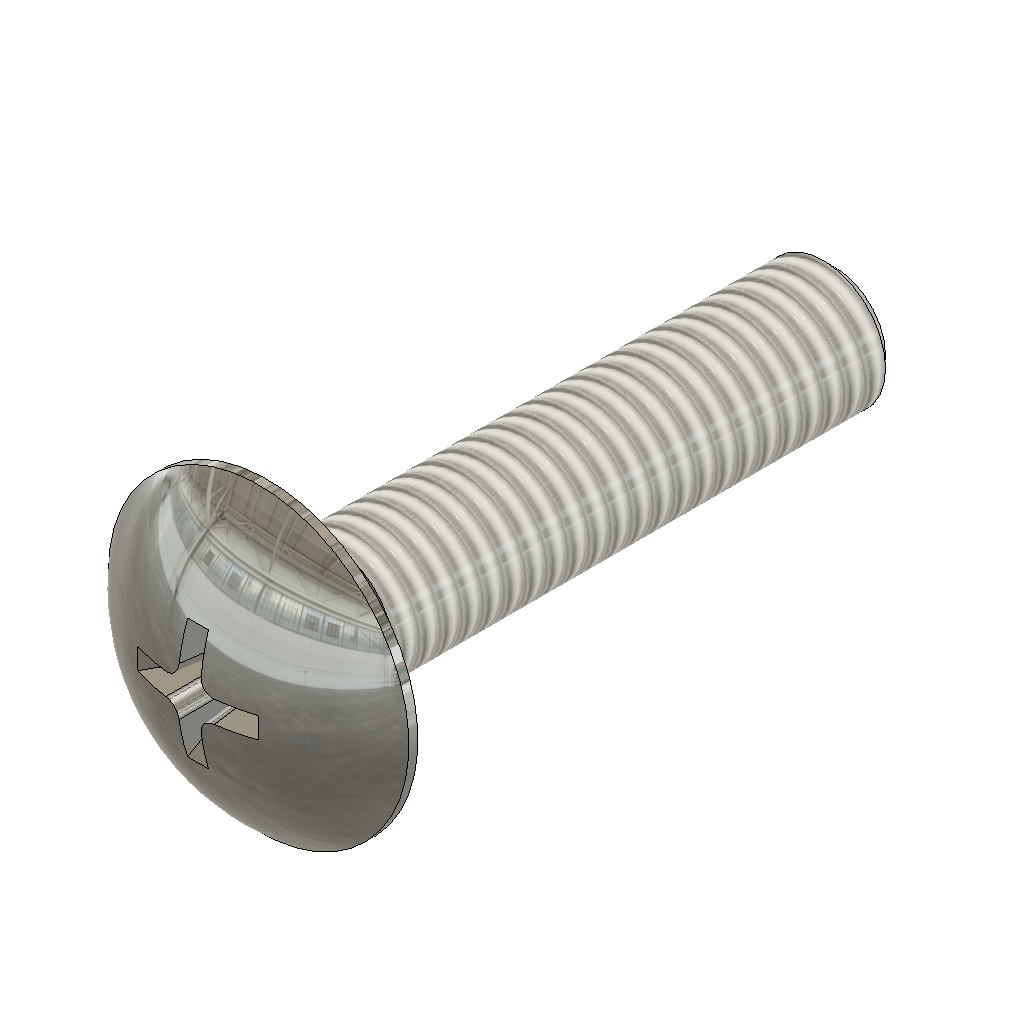
SdvxPanel (Assembly) (Autodesk Fusion 360 archive; units mm, degrees)
design "Truss Head Screw JIS B 1111 - M4.5x20 Steel 4.6 Chrome"
description: Truss Head Screw JIS B 1111 - M4.5x20
part number: THS JIS B 1111 - M4.5x20 Steel 4.6 Chrome
Autodesk Fusion 360 part; units mm, degrees
(part 1 of 4)
sketch "Sketch1" plane through (0, 0, 0) normal (0, 1, 0) x (1, 0, 0)
  line L0 (-2.25, 2.25) -> (-2.25, 20)
  line L1 (-2.25, 20) -> (0, 20)
  line L2 (0, 20) -> (0, -2.8)
  line L3 (-1.9125, 0) -> (-5.3, 0)
  line L4 (-5.3, 0) -> (-5.3, -0.3181)
  arc A0 (-5.3, -0.3181) -> (0, -2.8) centre (0, 4.1) ccw
  line L5 (-2.25, 2.25) -> (-1.9125, 2.25)
  line L6 (-1.9125, 2.25) -> (-1.9125, 0)
  dimension "d9" = 4.5
  dimension "d66" = 10.6
  dimension "d76" = 3.825
  dimension "d78" = 2.25
  dimension "d98" = 2.8
  dimension "d100" = 20
  constraint perpendicular L0 L1
  constraint perpendicular L0 L3
  constraint coincident origin L3
  constraint vertical L0
  constraint vertical L2
  constraint vertical L4
  constraint coincident L2 A0.centre
  constraint coincident L2.end A0.end
  constraint coincident L3.start L6.end
  constraint coincident origin L2
  measures "d78" distance of L3 L5
  measures "d98" distance of L3 L2.end
  measures "d100" distance of origin L1
revolve "Revolve1" add sketch "Sketch1" angle 360 about axis through (0, 0, -20) along (0, 0, 1) makes body 1
ref_plane "WorkPlane1" through (0, 0, 2.8) normal (0, 0, 1) x (1, 0, 0)
sketch "Sketch2" plane through (0, 0, 2.8) normal (0, 0, 1) x (1, 0, 0)
  line L0 (-0.3917, 0.3917) -> (-2.35, 0.3917)
  line L1 (-0.3917, -0.3917) -> (-2.35, -0.3917)
  line L2 (-2.35, 0.3917) -> (-2.35, -0.3917)
  line L3 (-0.3917, -0.3917) -> (-0.3917, -2.35)
  line L4 (-0.3917, -2.35) -> (0.3917, -2.35)
  line L5 (0.3917, -0.3917) -> (0.3917, -2.35)
  line L6 (0.3917, -0.3917) -> (2.35, -0.3917)
  line L7 (2.35, -0.3917) -> (2.35, 0.3917)
  line L8 (0.3917, 0.3917) -> (2.35, 0.3917)
  line L9 (0.3917, 0.3917) -> (0.3917, 2.35)
  line L10 (0.3917, 2.35) -> (-0.3917, 2.35)
  line L11 (-0.3917, 0.3917) -> (-0.3917, 2.35)
  dimension "d94" = 360
  dimension "d101" = 0.7833
  dimension "d102" = 4.7
  constraint horizontal L0
  constraint vertical L0.start L1.start
  constraint coincident L0.start L11.start
  constraint vertical L2
  measures "d101" distance of L0 L1
  measures "d102" distance of L2 L7
extrude "Extrude1" add sketch "Sketch2" against normal blind 2.53 draft -4 separate body makes body 2
draft "Draft1" angle -30 neutral plane through (0, 0, 2.8) pull (0, 0, 1) 4 faces at (-2.291, -0.0716, 1.9567) (0.0716, -2.291, 1.9567) (2.291, 0.0716, 1.9567) (0.0716, 2.291, 1.9567) on bodies 2
fillet "Fillet3" radius 0.47 4 edges at (-0.3032, 0.3032, 1.535) (0.3032, 0.3032, 1.535) (0.3032, -0.3032, 1.535) (-0.3032, -0.3032, 1.535) on bodies 2
combine "Combine1" operation cut target body 1 tool bodies 2
thread "Thread1" "ISO Metric profile 4.5 M4.5x0.75 M4.5x0.75 6g" major diameter 4.408 minor diameter 3.5525 pitch 0.75 angle 60 resizes the face on face at (-2.2388, 0.224, -8.1667) on bodies 1
sketch "Sketch6" plane through (0, 0, 0) normal (0, 1, 0) x (1, 0, 0)
  line L0 (-1.8, 20) -> (-2.295, 20)
  line L1 (-2.295, 20) -> (-2.295, 19.505)
  line L2 (-2.295, 19.505) -> (-1.8, 20)
  point P0 (0, 20)
  dimension "d83" = 45
  dimension "d85" = 2.295
  dimension "d103" = 0.495
  constraint horizontal L0
  constraint perpendicular L0 L1
  constraint coincident L0 P0
  measures "d83" angle of L1 L2
  measures "d85" distance of origin L1
  measures "d103" distance of L0 L1.end
revolve "Revolve3" cut sketch "Sketch6" angle 360 about axis through (0, 0, 1.75) along (0, 0, 1) bodies 1
equation "d9 = adsk_nomdia"
equation "adsk_nomlen = 20.00 mm"
equation "adsk_headh = 2.80 mm"
equation "adsk_headdia = 10.60 mm"
equation "adsk_nomdia = 4.50 mm"
equation "adsk_phildia = 4.70 mm"
equation "adsk_phildepth = 2.53 mm"
equation "d66 = adsk_headdia"
equation "d71 = adsk_headh"
equation "adsk_thrlen = 17.75 mm"
equation "d76 = adsk_nomdia * 0.85"
equation "d78 = adsk_nomlen - adsk_thrlen"
equation "d85 = adsk_nomdia * 0.51"
equation "adsk_ovalrad = 6.90 mm"
equation "d97 = adsk_phildia * 0.1"
equation "d98 = adsk_headh"
equation "d100 = adsk_nomlen"
equation "d101 = adsk_phildia / 6"
equation "d102 = adsk_phildia"
equation "d103 = adsk_nomdia * 0.1 + ( adsk_nomdia * 0.01 )"

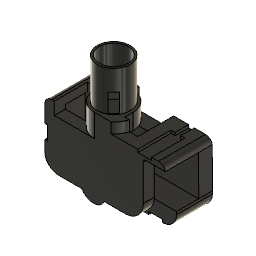
design "OBSA-LHS1F"
Autodesk Fusion 360 part; units mm, degrees
sketch "Sketch1" plane through (0, 0, 0) normal (0, 1, 0) x (1, 0, 0) in component "housing"
  line L0 (21.875, 5.25) -> (21.875, 6.25)
  line L1 (21.875, 11.25) -> (-21.875, -11.25) construction
  line L2 (-21.875, 11.25) -> (21.875, -11.25) construction
  line L3 (-0.275, 11.25) -> (-0.275, 13.75) construction
  line L4 (-0.275, 13.75) -> (-8.375, 13.75) construction
  line L5 (-8.375, 13.75) -> (-8.375, 11.25) construction
  arc A0 (21.875, 6.25) -> (16.875, 11.25) centre (16.875, 6.25) ccw
  arc A1 (-16.875, 11.25) -> (-21.875, 6.25) centre (-16.875, 6.25) ccw
  line L6 (-18.375, -11.25) -> (-18.375, -6.75)
  arc A2 (-21.875, -8.75) -> (-19.375, -11.25) centre (-19.375, -8.75) ccw
  line L7 (-18.375, -6.75) -> (-6.875, -6.75)
  line L8 (-6.875, -6.75) -> (-6.875, -11.25)
  line L9 (21.875, 5.25) -> (13.8245, 5.25)
  arc A3 (19.375, -11.25) -> (21.8245, -9.25) centre (19.375, -8.75) ccw
  line L10 (21.8245, -9.25) -> (14.8245, -9.25)
  line L11 (13.8245, -8.25) -> (13.8245, 5.25)
  line L12 (-19.375, -11.25) -> (-18.375, -11.25)
  arc A4 (-0.275, 11.25) -> (-8.375, 11.25) centre (-4.325, 9.2195) ccw
  line L13 (-8.375, 11.25) -> (-16.875, 11.25)
  line L14 (16.8245, -11.25) -> (16.8245, -10.25)
  line L15 (16.8245, -10.25) -> (11.8245, -10.25)
  line L16 (11.8245, -10.25) -> (11.8245, -11.25)
  line L17 (7.8245, -11.25) -> (11.8245, -11.25)
  line L18 (16.8245, -11.25) -> (19.375, -11.25)
  line L19 (-21.875, -2.5) -> (-20.875, -2.5)
  line L20 (-20.875, -2.5) -> (-20.875, 2.5)
  line L21 (-20.875, 2.5) -> (-21.875, 2.5)
  line L22 (-21.875, 6.25) -> (-21.875, 2.5)
  line L23 (-21.875, -2.5) -> (-21.875, -8.75)
  line L24 (-21.4773, 11.25) -> (-21.4773, 0) construction
  line L25 (-20.875, 0) -> (-22.0795, 0) construction
  line L26 (-21.4773, -11.25) -> (-21.4773, 0) construction
  arc A5 (13.8245, -8.25) -> (14.8245, -9.25) centre (14.8245, -8.25) ccw
  line L27 (11.8245, 11.25) -> (11.8245, 10.25)
  line L28 (11.8245, 10.25) -> (16.8245, 10.25)
  line L29 (16.8245, 10.25) -> (16.8245, 11.25)
  line L30 (16.875, 11.25) -> (16.8245, 11.25)
  line L31 (11.8245, 11.25) -> (-0.275, 11.25)
  line L32 (7.8245, -11.25) -> (7.8245, -6.75)
  line L33 (7.8245, -6.75) -> (-6.875, -6.75)
  line L34 (7.8245, -11.25) -> (-6.875, -11.25)
  line L35 (-6.875, -11.25) -> (-18.375, -11.25)
  point P0 (-4.325, 13.75)
  point P1 (13.8245, -9.25)
  dimension "d1" = 43.75
  dimension "d2" = 22.5
  dimension "d4" = 8.1
  dimension "d5" = 2.5
  dimension "d6" = 13.5
  dimension "d13" = 5
  dimension "d14" = 5
  dimension "d15" = 4.5
  dimension "d16" = 2.5
  dimension "d18" = 3.5
  dimension "d19" = 6
  dimension "d21" = 2.5
  dimension "d22" = 2
  dimension "d23" = 8
  dimension "d24" = 1
  dimension "d25" = 5
  dimension "d26" = 5
  dimension "d27" = 5
  dimension "d28" = 1
  dimension "d29" = 1
  dimension "d38" = 4.5
  dimension "d39" = 14
  dimension "d69" = 15
  constraint horizontal L30
  constraint perpendicular L22 L30
  constraint parallel L12 L30
  constraint parallel L0 L22
  constraint coincident L1 origin
  constraint coincident L2 origin
  constraint vertical L3
  constraint horizontal L4
  constraint vertical L5
  constraint coincident L5.end L30
  constraint midpoint L4 P0
  constraint coincident P0 A4
  constraint coincident L1.start L0
  constraint coincident L1.start L30
  constraint tangent L0 A0
  constraint tangent A0 L30
  constraint coincident L2.start L22
  constraint coincident L2.start L30
  constraint tangent A1 L22
  constraint tangent A1 L30
  constraint perpendicular L6 L12
  constraint coincident L1.end L22
  constraint coincident L1.end L12
  constraint tangent A2 L22
  constraint tangent A2 L12
  constraint coincident L8.end L12
  constraint perpendicular L8 L12
  constraint horizontal L7
  constraint perpendicular L0 L9
  constraint coincident L2.end L0
  constraint coincident L2.end L12
  constraint tangent L0 A3
  constraint tangent A3 L12
  constraint horizontal L10
  constraint coincident L9 L11.end
  constraint perpendicular L9 L11
  constraint collinear L12 L17
  constraint collinear L13 L30
  constraint coincident L14.start L17
  constraint perpendicular L14 L17
  constraint perpendicular L14 L15
  constraint perpendicular L16 L17
  constraint collinear L17 L18
  constraint coincident L19.start L22
  constraint perpendicular L19 L22
  constraint perpendicular L19 L20
  constraint perpendicular L21 L22
  constraint collinear L22 L23
  constraint coincident L13 L24.start
  constraint perpendicular L13 L24
  constraint midpoint L20 L25.start
  constraint perpendicular L20 L25
  constraint midpoint L24.end L25
  constraint coincident L12 L26.start
  constraint perpendicular L12 L26
  constraint midpoint L25 L24.end
  constraint equal L24 L26
  constraint coincident P1 L10
  constraint coincident P1 L11
  constraint tangent L10 A5
  constraint tangent L11 A5
  constraint coincident L27.start L30
  constraint perpendicular L27 L30
  constraint perpendicular L27 L28
  constraint perpendicular L29 L30
  constraint equal L15 L28
  constraint equal L14 L27
  constraint collinear L16 L27
  constraint collinear L30 L31
  constraint perpendicular L17 L32
  constraint perpendicular L8 L34
  measures "d1" distance of L1.end L2.end
  measures "d2" distance of L2.start L1.end
  measures "d4" distance of L5.end L3.start
  measures "d5" distance of L5.end L4.end
  measures "d6" distance of L5 L22
  measures "d13" radius of A0
  measures "d14" radius of A1
  measures "d15" distance of L6.start L6.end
  measures "d16" radius of A2
  measures "d18" distance of L6 L22
  measures "d19" distance of L9 L30
  measures "d21" radius of A3
  measures "d22" distance of L10 L12
  measures "d23" distance of A3.end P1
  measures "d24" distance of L14.start L14.end
  measures "d25" distance of A3.end L14
  measures "d26" distance of L14.end L15.end
  measures "d27" distance of L19.end L20.end
  measures "d28" distance of L19.start L19.end
  measures "d29" radius of A5
  measures "d38" distance of L17.start L32.end
  measures "d39" distance of A3.end L32
  measures "d69" distance of L8 L23
extrude "Extrude1" add sketch "Sketch1" along normal mid plane 8 contours L0 A0 A1 L6 A2 L7 L9 A3 L10 L11 L12 A4 L13 L14 L15 L16 L17 L18 L19 L20 L21 L22 L23 A5 L27 L28 L29 L30 L31 L32 L33 in component "housing"
sketch "Sketch2" plane through (0, -4, 0) normal (0, -1, 0) x (1, 0, 0) in component "housing"
  line L0 (16.8245, -11.25) -> (16.875, -11.25)
  line L1 (21.875, -6.25) -> (21.875, -5.25)
  line L2 (19.375, 11.25) -> (16.8245, 11.25)
  line L3 (-21.875, -2.5) -> (-21.875, -6.25)
  arc A0 (-8.375, -11.25) -> (-0.275, -11.25) centre (-4.325, -9.2195) ccw
  arc A1 (-8.375, -11.25) -> (-0.275, -11.25) centre (-4.325, -9.2195) ccw
  line L4 (-21.875, 2.5) -> (-20.875, 2.5)
  line L5 (-20.875, 2.5) -> (-20.875, -2.5)
  line L6 (-20.875, -2.5) -> (-21.875, -2.5)
  arc A2 (-21.875, -6.25) -> (-16.875, -11.25) centre (-16.875, -6.25) ccw
  arc A3 (16.875, -11.25) -> (21.875, -6.25) centre (16.875, -6.25) ccw
  line L7 (21.875, -5.25) -> (13.8245, -5.25)
  line L8 (13.8245, -5.25) -> (13.8245, 8.25)
  line L9 (14.8245, 9.25) -> (21.8245, 9.25)
  arc A4 (21.8245, 9.25) -> (19.375, 11.25) centre (19.375, 8.75) ccw
  line L10 (16.8245, 11.25) -> (16.8245, 10.25)
  line L11 (16.8245, 10.25) -> (11.8245, 10.25)
  line L12 (11.8245, 10.25) -> (11.8245, 11.25)
  line L13 (11.8245, 11.25) -> (7.8245, 11.25)
  line L14 (7.8245, 6.75) -> (-18.375, 6.75)
  line L15 (-18.375, 6.75) -> (-18.375, 11.25)
  line L16 (-18.375, 11.25) -> (-19.375, 11.25)
  arc A5 (-19.375, 11.25) -> (-21.875, 8.75) centre (-19.375, 8.75) ccw
  line L17 (-21.875, 8.75) -> (-21.875, 2.5)
  arc A6 (14.8245, 9.25) -> (13.8245, 8.25) centre (14.8245, 8.25) ccw
  circle A7 centre (7.3245, -4.75) radius 6.5
  line L18 (13.8245, -4.75) -> (13.8245, -5.25)
  line L19 (11.8245, -11.25) -> (11.8245, -10.25)
  line L20 (11.8245, -10.25) -> (16.8245, -10.25)
  line L21 (16.8245, -10.25) -> (16.8245, -11.25)
  line L22 (-16.875, -11.25) -> (-8.375, -11.25)
  line L23 (-0.275, -11.25) -> (11.8245, -11.25)
  line L24 (7.8245, 11.25) -> (7.8245, 6.75)
  line L25 (7.8245, 11.25) -> (-6.875, 11.25)
  line L26 (-6.875, 6.75) -> (-6.875, 11.25)
  dimension "d30" = 13
  dimension "d84" = 0.5
  constraint tangent L8 A7
  constraint coincident A7 L18.start
  constraint perpendicular L7 L18
  constraint collinear L8 L18
  constraint coincident L7.end L8.start
  constraint tangent A7 L23
  measures "d30" diameter of A7
extrude "Extrude2" add sketch "Sketch2" along normal blind 4 contours L2 L3 A0 A1 L4 L5 L6 A2 L8 L9 A4 L10 L11 L12 L13 L14 L15 L16 A5 L17 A6 A7 L22 L23 L24 | A7 | L14 L24 L25 L26 in component "housing"
sketch "Sketch3" plane through (0, 4, 0) normal (0, 1, 0) x (1, 0, 0) in component "housing"
  line L0 (21.8245, -9.25) -> (21.875, 5.25)
  line L1 (7.8245, -11.25) -> (-18.375, -11.25)
  line L2 (16.8245, -11.25) -> (15.3245, -11.25)
  line L3 (15.3245, -11.25) -> (15.3245, -10.25)
  line L4 (11.8245, -11.25) -> (13.3245, -11.25)
  line L5 (13.3245, -11.25) -> (13.3245, -10.25)
  line L6 (16.8245, 11.25) -> (15.3245, 11.25)
  line L7 (15.3245, 11.25) -> (15.3245, 10.2907)
  line L8 (11.8245, 11.25) -> (13.3245, 11.25)
  line L9 (13.3245, 11.25) -> (13.3245, 10.2452)
  line L10 (-21.875, -2.5) -> (-21.875, -1)
  line L11 (-21.875, -1) -> (-20.875, -1)
  line L12 (-21.875, 2.5) -> (-21.875, 1)
  line L13 (-21.875, 1) -> (-20.875, 1)
  line L14 (7.8245, -11.25) -> (11.8245, -11.25)
  line L15 (11.8245, -11.25) -> (11.8245, -10.25)
  line L16 (11.8245, -10.25) -> (16.8245, -10.25)
  line L17 (16.8245, -10.25) -> (16.8245, -11.25)
  line L18 (16.8245, -11.25) -> (19.375, -11.25)
  arc A0 (19.375, -11.25) -> (21.8245, -9.25) centre (19.375, -8.75) ccw
  line L19 (21.8245, -9.25) -> (14.8245, -9.25)
  arc A1 (13.8245, -8.25) -> (14.8245, -9.25) centre (14.8245, -8.25) ccw
  line L20 (13.8245, -8.25) -> (13.8245, 5.25)
  line L21 (13.8245, 5.25) -> (21.875, 5.25)
  line L22 (21.875, 5.25) -> (21.875, 6.25)
  arc A2 (21.875, 6.25) -> (16.875, 11.25) centre (16.875, 6.25) ccw
  line L23 (16.875, 11.25) -> (16.8245, 11.25)
  line L24 (16.8245, 11.25) -> (16.8245, 10.25)
  line L25 (16.8245, 10.25) -> (11.8245, 10.25)
  line L26 (11.8245, 10.25) -> (11.8245, 11.25)
  line L27 (11.8245, 11.25) -> (-0.275, 11.25)
  arc A3 (-0.275, 11.25) -> (-8.375, 11.25) centre (-4.325, 9.2195) ccw
  line L28 (-8.375, 11.25) -> (-16.875, 11.25)
  arc A4 (-16.875, 11.25) -> (-21.875, 6.25) centre (-16.875, 6.25) ccw
  line L29 (-21.875, 6.25) -> (-21.875, 2.5)
  line L30 (-21.875, 2.5) -> (-20.875, 2.5)
  line L31 (-20.875, 2.5) -> (-20.875, -2.5)
  line L32 (-20.875, -2.5) -> (-21.875, -2.5)
  line L33 (-21.875, -2.5) -> (-21.875, -8.75)
  arc A5 (-21.875, -8.75) -> (-19.375, -11.25) centre (-19.375, -8.75) ccw
  line L34 (-19.375, -11.25) -> (-18.375, -11.25)
  line L35 (-18.375, -11.25) -> (-18.375, -6.75)
  line L36 (-18.375, -6.75) -> (7.8245, -6.75)
  line L37 (7.8245, -6.75) -> (7.8245, -11.25)
  line L38 (-6.875, -6.75) -> (-6.875, -11.25)
  dimension "d35" = 2
  dimension "d36" = 2
  dimension "d37" = 2
  constraint equal L2 L4
  constraint equal L6 L8
  constraint equal L10 L12
  constraint coincident L0.end L21.end
  constraint coincident L0.start A0.end
  constraint coincident L2.start L17.end
  constraint coincident L4.start L14.end
  constraint coincident L3.end L16
  constraint perpendicular L3 L16
  constraint vertical L5
  constraint horizontal L2
  constraint horizontal L4
  constraint horizontal L1
  constraint coincident L1.start L14.start
  constraint coincident L1.end L34.end
  constraint coincident L11.end L31
  constraint perpendicular L11 L31
  constraint coincident L10.start L32.end
  constraint vertical L10
  constraint vertical L12
  constraint coincident L13.end L31
  constraint horizontal L13
  constraint coincident L12.start L29.end
  constraint coincident L8.start L26.end
  constraint coincident L6.start L23.end
  constraint vertical L7
  constraint horizontal L6
  constraint horizontal L8
  measures "d35" distance of L2.end L4.end
  measures "d36" distance of L7 L9
  measures "d37" distance of L10.end L12.end
extrude "Extrude3" add sketch "Sketch3" along normal blind 5 contours L0 L19 A1 L20 L21 | L14 L15 L16 L17 L18 A0 L19 A1 L20 L21 L22 A2 L23 L24 L25 L26 L27 A3 L28 A4 L29 L30 L31 L32 L33 A5 L34 L35 L36 L37 | L2 L3 L16 L17 | L4 L5 L15 L16 | L8 L9 L25 L26 | L1 L35 L36 L38 | L12 L13 L30 L31 | L10 L11 L31 L32 in component "housing"
sketch "Sketch4" plane through (0, 0, 11.25) normal (0, 0, 1) x (-1, 0, 0) in component "housing"
  line L0 (-11.8245, 8) -> (-11.8245, -4)
  line L1 (-13.3245, -9) -> (-7.8245, -9)
  line L2 (-7.8245, -9) -> (-7.8245, 4)
  line L3 (-7.8245, 4) -> (6.875, 4)
  line L4 (6.875, 4) -> (6.875, 8)
  line L5 (6.875, 8) -> (-11.8245, 8)
  circle A0 centre (3.875, 1) radius 6
  circle A1 centre (3.875, 1) radius 7
  line L6 (10.875, 10.5333) -> (10.875, -12) construction
  line L7 (21.875, 8) -> (21.875, -9)
  line L8 (18.375, -4) -> (6.875, -4)
  line L9 (-7.8245, 4) -> (6.875, 4)
  line L10 (-11.8245, 8) -> (6.875, 8)
  line L11 (6.875, 4) -> (6.875, 8)
  line L12 (-11.8245, 8) -> (-11.8245, -4)
  line L13 (-7.8245, -9) -> (-7.8245, 4)
  line L14 (18.375, 8) -> (18.375, -4)
  line L15 (6.875, -9) -> (19.375, -9)
  line L16 (19.375, -9) -> (19.375, 8)
  line L17 (19.375, 8) -> (18.375, 8)
  line L18 (10.875, 1) -> (10.875, -4)
  line L19 (3.875, -8.25) -> (3.875, -6)
  arc A2 (-2.1717, 8) -> (-4.875, 4) centre (3.875, 1) ccw
  arc A3 (3.875, -8.25) -> (11.6572, -4) centre (3.875, 1) ccw
  line L20 (-4.875, 4) -> (-2.4496, 4)
  line L21 (-2.1717, 8) -> (3.875, 8)
  line L22 (-2.1717, 8) -> (3.875, 8)
  line L23 (10.875, -4) -> (11.6572, -4)
  line L24 (-3.125, 4) -> (-3.125, 1)
  circle A4 centre (3.875, 1) radius 5.25
  line L25 (17.875, -13) -> (-10.3827, 15.2577) construction
  line L26 (17.875, -13) -> (57.8375, -13) construction
  line L27 (-1.2936, 4.0473) -> (-3.5496, 6.3033)
  line L28 (-3.5496, 6.3033) -> (-1.4283, 8.4246)
  line L29 (-1.4283, 8.4246) -> (0.8277, 6.1686)
  line L30 (-2.0305, 3.5798) -> (1.1775, 6.7878) construction
  line L31 (-7.6794, -10.5544) -> (19.2768, 16.4018) construction
  line L32 (6.9223, -4.1686) -> (9.1783, -6.4246)
  line L33 (11.2996, -4.3033) -> (9.0436, -2.0473)
  line L34 (9.1783, -6.4246) -> (11.2996, -4.3033)
  line L35 (-11.8245, -4) -> (-13.3245, -4)
  line L36 (-13.3245, -4) -> (-13.3245, -9)
  line L37 (18.375, -4) -> (6.875, -4)
  line L38 (6.875, -4) -> (6.875, -9)
  dimension "d42" = 12
  dimension "d43" = 14
  dimension "d44" = 18.5
  dimension "d45" = 11
  dimension "d48" = 10.5
  dimension "d58" = 135
  dimension "d63" = 1.5
  dimension "d64" = 1.5
  dimension "d65" = 3
  constraint concentric A0 A1
  constraint tangent L5 A1
  constraint concentric A1 A2
  constraint vertical L6
  constraint tangent A1 L6
  constraint coincident L8 A3.end
  constraint coincident L5 A2.start
  constraint coincident L6 L18.start
  constraint coincident A1 L18.start
  constraint coincident L6 L18.end
  constraint coincident L8 L18.end
  constraint coincident L19.start A2
  constraint coincident A1 L19.end
  constraint parallel L18 L19
  constraint collinear A0.centre L19.start L19.end
  constraint coincident L3 A2.end
  constraint concentric A2 A3
  constraint coincident L3 L20.end
  constraint coincident A1 L20.end
  constraint coincident A1 L21.end
  constraint coincident L10 L21.end
  constraint coincident L9 L24.start
  constraint perpendicular L20 L24
  constraint tangent A1 L24
  constraint coincident A1 L24.end
  constraint concentric A0 A4
  constraint horizontal L26
  constraint coincident A0.centre L25
  constraint perpendicular L25 L28
  constraint perpendicular L28 L29
  constraint parallel L25 L27
  constraint perpendicular L29 L30
  constraint perpendicular L25 L31
  constraint coincident A0.centre L31
  constraint symmetric L27.start L31 L32.start
  constraint symmetric L27.end L31 L32.end
  constraint symmetric L28.end L31 L33.start
  constraint symmetric L29.end L31 L33.end
  constraint tangent A0 L30
  constraint coincident A0 L27.start
  constraint coincident A0 L29.end
  measures "d42" diameter of A0
  measures "d43" diameter of A1
  measures "d44" diameter of A2
  measures "d45" distance of L6 L7
  measures "d48" diameter of A4
  measures "d58" angle of L25 L26
  measures "d63" distance of L25 L27
  measures "d64" distance of L25 L29
  measures "d65" distance of L28 L30
extrude "Extrude4" cut sketch "Sketch4" against normal blind 4.5 contours L3 L5 A1 L9 L10 A2 L20 L21 L22 L27 L28 | L5 A1 L10 L21 L22 L27 L28 L29 | L5 A1 L10 L21 L22 L29 | L3 A1 L9 L20 L24 | L4 A0 A1 L11 L29 | A0 A1 L27 L29 | L3 A0 A1 L9 L27 | L3 A0 A1 L9 L38 | L4 A0 A1 L11 L33 | L3 L4 A0 L9 L11 A4 | L3 L4 A0 L8 L9 L11 A4 L37 L38 | A1 L19 A3 L38 | A1 L18 L33 | L3 L4 L9 L11 A4 | L3 L4 L9 L11 A4 | A0 L8 L37 L38 | A0 A1 L32 L38 | A1 L8 A3 L23 L32 L33 L34 L37 L38 | A1 L8 L18 L33 L37 | A0 A1 L8 L33 L37 | A0 A1 L8 L32 L37 | A1 L8 L23 L32 L33 L34 L37 in component "housing"
extrude "Extrude5" add sketch "Sketch4" along normal blind -4.5 and the other way blind -3.75 contours L3 L5 A1 L9 L10 A2 L20 L21 L22 L27 L28 | L5 A1 L10 L21 L22 L27 L28 L29 | L5 A1 L10 L21 L22 L29 | L3 A1 L9 L20 L24 | L4 A0 A1 L11 L29 | A0 A1 L27 L29 | L3 A0 A1 L9 L27 | L3 A0 A1 L9 L38 | L4 A0 A1 L11 L33 | L3 L4 A0 L9 L11 A4 | L3 L4 A0 L8 L9 L11 A4 L37 L38 | A1 L19 A3 L38 | L3 L4 L9 L11 A4 | L3 L4 L9 L11 A4 | A0 L8 L37 L38 | A0 A1 L32 L38 | A1 L8 A3 L23 L32 L33 L34 L37 L38 | A0 A1 L8 L33 L37 | A0 A1 L8 L32 L37 | A1 L8 L23 L32 L33 L34 L37 in component "housing"
extrude "Extrude6" cut sketch "Sketch4" against normal blind 4.5 contours L4 L5 A1 L10 L11 in component "housing"
extrude "Extrude7" add sketch "Sketch4" along normal blind 14.5 from surface at 3.75 contours L3 L4 A0 L9 L11 A4 | L3 L4 A0 L8 L9 L11 A4 L37 L38 | A0 L8 L37 L38 in component "housing"
extrude "Extrude8" add sketch "Sketch4" along normal blind 4.5 from surface at 6.25 contours L5 L10 L21 L22 L28 L29 | L5 A1 L10 L21 L22 L27 L28 L29 | A0 A1 L27 L29 | A1 L8 L18 L33 L37 | A0 A1 L8 L33 L37 | L8 L18 L23 L33 L37 | A0 A1 L8 L32 L37 | A1 L8 L23 L32 L33 L34 L37 in component "housing"
sketch "Sketch5" plane through (0, 9, 0) normal (0, 1, 0) x (-1, 0, 0) in component "housing"
  line L0 (-15.3245, 10.25) -> (-15.3245, 11.25)
  line L1 (-15.3245, 11.25) -> (-19.375, 11.25)
  arc A0 (-19.375, 11.25) -> (-21.8245, 9.25) centre (-19.375, 8.75) ccw
  line L2 (-21.8245, 9.25) -> (-21.875, -5.25)
  line L3 (-21.875, -5.25) -> (-21.875, -6.25)
  arc A1 (-21.875, -6.25) -> (-16.875, -11.25) centre (-16.875, -6.25) ccw
  line L4 (-16.875, -11.25) -> (-16.8245, -11.25)
  line L5 (-16.8245, -11.25) -> (-16.8245, -10.25)
  line L6 (-16.8245, -10.25) -> (-13.3245, -10.25)
  line L7 (-13.3245, -10.25) -> (-13.3245, -11.25)
  line L8 (-13.3245, -11.25) -> (0.275, -11.25)
  arc A2 (0.275, -11.25) -> (8.375, -11.25) centre (4.325, -9.2195) ccw
  line L9 (8.375, -11.25) -> (16.875, -11.25)
  arc A3 (16.875, -11.25) -> (21.875, -6.25) centre (16.875, -6.25) ccw
  line L10 (21.875, -6.25) -> (21.875, -1)
  line L11 (21.875, -1) -> (20.875, -1)
  line L12 (20.875, -1) -> (20.875, 1)
  line L13 (20.875, 1) -> (21.875, 1)
  line L14 (21.875, 1) -> (21.875, 2.5)
  line L15 (21.875, 2.5) -> (21.875, 8.75)
  arc A4 (21.875, 8.75) -> (19.375, 11.25) centre (19.375, 8.75) ccw
  line L16 (19.375, 11.25) -> (6.875, 11.25)
  line L17 (6.875, 11.25) -> (6.875, 6.75)
  line L18 (6.875, 6.75) -> (-7.8245, 6.75)
  line L19 (-7.8245, 6.75) -> (-7.8245, 11.25)
  line L20 (-7.8245, 11.25) -> (-13.3245, 11.25)
  line L21 (-13.3245, 11.25) -> (-13.3245, 10.25)
  line L22 (-13.3245, 10.25) -> (-15.3245, 10.25)
  line L23 (11.375, 11.25) -> (11.375, -11.25) construction
  line L24 (-11.8245, 11.25) -> (-11.8245, -11.25) construction
  line L25 (-3.6673, -8.472) -> (-3.4217, -8.4393)
  spline S0 degree 2 poles (-3.4217, -8.4393) (-3.3794, -8.648) (-3.2785, -8.7408) knots 0 0 0 1 1 1
  spline S1 degree 2 poles (-3.2785, -8.7408) (-3.1762, -8.8322) (-3.0302, -8.8322) knots 0 0 0 1 1 1
  spline S2 degree 2 poles (-3.0302, -8.8322) (-2.8569, -8.8322) (-2.7382, -8.7121) knots 0 0 0 1 1 1
  spline S3 degree 2 poles (-2.7382, -8.7121) (-2.6182, -8.5921) (-2.6182, -8.4147) knots 0 0 0 1 1 1
  spline S4 degree 2 poles (-2.6182, -8.4147) (-2.6182, -8.2456) (-2.7287, -8.1364) knots 0 0 0 1 1 1
  spline S5 degree 2 poles (-2.7287, -8.1364) (-2.8392, -8.0259) (-3.0097, -8.0259) knots 0 0 0 1 1 1
  spline S6 degree 2 poles (-3.0097, -8.0259) (-3.0793, -8.0259) (-3.183, -8.0532) knots 0 0 0 1 1 1
  line L26 (-3.183, -8.0532) -> (-3.1557, -7.8377)
  spline S7 degree 2 poles (-3.1557, -7.8377) (-3.1311, -7.8404) (-3.1161, -7.8404) knots 0 0 0 1 1 1
  spline S8 degree 2 poles (-3.1161, -7.8404) (-2.9592, -7.8404) (-2.8337, -7.7585) knots 0 0 0 1 1 1
  spline S9 degree 2 poles (-2.8337, -7.7585) (-2.7082, -7.6767) (-2.7082, -7.5061) knots 0 0 0 1 1 1
  spline S10 degree 2 poles (-2.7082, -7.5061) (-2.7082, -7.3711) (-2.7996, -7.2824) knots 0 0 0 1 1 1
  spline S11 degree 2 poles (-2.7996, -7.2824) (-2.891, -7.1937) (-3.0356, -7.1937) knots 0 0 0 1 1 1
  spline S12 degree 2 poles (-3.0356, -7.1937) (-3.1789, -7.1937) (-3.2744, -7.2838) knots 0 0 0 1 1 1
  spline S13 degree 2 poles (-3.2744, -7.2838) (-3.3699, -7.3738) (-3.3972, -7.5539) knots 0 0 0 1 1 1
  line L27 (-3.3972, -7.5539) -> (-3.6427, -7.5102)
  spline S14 degree 2 poles (-3.6427, -7.5102) (-3.5977, -7.2633) (-3.4381, -7.1282) knots 0 0 0 1 1 1
  spline S15 degree 2 poles (-3.4381, -7.1282) (-3.2785, -6.9918) (-3.0411, -6.9918) knots 0 0 0 1 1 1
  spline S16 degree 2 poles (-3.0411, -6.9918) (-2.8774, -6.9918) (-2.7396, -7.0628) knots 0 0 0 1 1 1
  spline S17 degree 2 poles (-2.7396, -7.0628) (-2.6018, -7.1323) (-2.5295, -7.2538) knots 0 0 0 1 1 1
  spline S18 degree 2 poles (-2.5295, -7.2538) (-2.4558, -7.3752) (-2.4558, -7.5116) knots 0 0 0 1 1 1
  spline S19 degree 2 poles (-2.4558, -7.5116) (-2.4558, -7.6412) (-2.5254, -7.7476) knots 0 0 0 1 1 1
  spline S20 degree 2 poles (-2.5254, -7.7476) (-2.595, -7.854) (-2.7314, -7.9168) knots 0 0 0 1 1 1
  spline S21 degree 2 poles (-2.7314, -7.9168) (-2.5541, -7.9577) (-2.4558, -8.0873) knots 0 0 0 1 1 1
  spline S22 degree 2 poles (-2.4558, -8.0873) (-2.3576, -8.2156) (-2.3576, -8.4093) knots 0 0 0 1 1 1
  spline S23 degree 2 poles (-2.3576, -8.4093) (-2.3576, -8.6712) (-2.5486, -8.854) knots 0 0 0 1 1 1
  spline S24 degree 2 poles (-2.5486, -8.854) (-2.7396, -9.0355) (-3.0315, -9.0355) knots 0 0 0 1 1 1
  spline S25 degree 2 poles (-3.0315, -9.0355) (-3.2948, -9.0355) (-3.4695, -8.8786) knots 0 0 0 1 1 1
  spline S26 degree 2 poles (-3.4695, -8.8786) (-3.6427, -8.7217) (-3.6673, -8.472) knots 0 0 0 1 1 1
  line L28 (-1.6659, -9) -> (-2.1966, -7)
  line L29 (-2.1966, -7) -> (-1.9251, -7)
  line L30 (-1.9251, -7) -> (-1.6209, -8.3111)
  spline S27 degree 2 poles (-1.6209, -8.3111) (-1.5718, -8.5171) (-1.5363, -8.7203) knots 0 0 0 1 1 1
  spline S28 degree 2 poles (-1.5363, -8.7203) (-1.4599, -8.3997) (-1.4463, -8.3506) knots 0 0 0 1 1 1
  line L31 (-1.4463, -8.3506) -> (-1.0657, -7)
  line L32 (-1.0657, -7) -> (-0.7464, -7)
  line L33 (-0.7464, -7) -> (-0.4599, -8.0123)
  spline S29 degree 2 poles (-0.4599, -8.0123) (-0.3521, -8.3888) (-0.3044, -8.7203) knots 0 0 0 1 1 1
  spline S30 degree 2 poles (-0.3044, -8.7203) (-0.2662, -8.5307) (-0.2048, -8.2851) knots 0 0 0 1 1 1
  line L34 (-0.2048, -8.2851) -> (0.109, -7)
  line L35 (0.109, -7) -> (0.375, -7)
  line L36 (0.375, -7) -> (-0.1734, -9)
  line L37 (-0.1734, -9) -> (-0.4285, -9)
  line L38 (-0.4285, -9) -> (-0.8501, -7.4761)
  spline S31 degree 2 poles (-0.8501, -7.4761) (-0.9033, -7.2851) (-0.9129, -7.2415) knots 0 0 0 1 1 1
  spline S32 degree 2 poles (-0.9129, -7.2415) (-0.9442, -7.3793) (-0.9715, -7.4761) knots 0 0 0 1 1 1
  line L39 (-0.9715, -7.4761) -> (-1.3958, -9)
  line L40 (-1.3958, -9) -> (-1.6659, -9)
  line L41 (-11.8245, -9) -> (-11.8245, -7)
  line L42 (-11.8245, -7) -> (-11.5598, -7)
  line L43 (-11.5598, -7) -> (-11.5598, -8.764)
  line L44 (-11.5598, -8.764) -> (-10.5748, -8.764)
  line L45 (-10.5748, -8.764) -> (-10.5748, -9)
  line L46 (-10.5748, -9) -> (-11.8245, -9)
  line L47 (-10.2539, -9) -> (-10.2539, -7)
  line L48 (-10.2539, -7) -> (-9.8555, -7)
  line L49 (-9.8555, -7) -> (-9.3821, -8.4161)
  spline S33 degree 2 poles (-9.3821, -8.4161) (-9.3167, -8.6139) (-9.2866, -8.7121) knots 0 0 0 1 1 1
  spline S34 degree 2 poles (-9.2866, -8.7121) (-9.2525, -8.603) (-9.1802, -8.3915) knots 0 0 0 1 1 1
  line L50 (-9.1802, -8.3915) -> (-8.7014, -7)
  line L51 (-8.7014, -7) -> (-8.3453, -7)
  line L52 (-8.3453, -7) -> (-8.3453, -9)
  line L53 (-8.3453, -9) -> (-8.6004, -9)
  line L54 (-8.6004, -9) -> (-8.6004, -7.3261)
  line L55 (-8.6004, -7.3261) -> (-9.1816, -9)
  line L56 (-9.1816, -9) -> (-9.4203, -9)
  line L57 (-9.4203, -9) -> (-9.9988, -7.2974)
  line L58 (-9.9988, -7.2974) -> (-9.9988, -9)
  line L59 (-9.9988, -9) -> (-10.2539, -9)
  line L60 (-7.9043, -9) -> (-7.9043, -7)
  line L61 (-7.9043, -7) -> (-7.1499, -7)
  spline S35 degree 2 poles (-7.1499, -7) (-6.9507, -7) (-6.8457, -7.0191) knots 0 0 0 1 1 1
  spline S36 degree 2 poles (-6.8457, -7.0191) (-6.6983, -7.0437) (-6.5987, -7.1132) knots 0 0 0 1 1 1
  spline S37 degree 2 poles (-6.5987, -7.1132) (-6.4991, -7.1814) (-6.4391, -7.3056) knots 0 0 0 1 1 1
  spline S38 degree 2 poles (-6.4391, -7.3056) (-6.3777, -7.4297) (-6.3777, -7.5784) knots 0 0 0 1 1 1
  spline S39 degree 2 poles (-6.3777, -7.5784) (-6.3777, -7.8336) (-6.5401, -8.0109) knots 0 0 0 1 1 1
  spline S40 degree 2 poles (-6.5401, -8.0109) (-6.7024, -8.1869) (-7.1267, -8.1869) knots 0 0 0 1 1 1
  line L62 (-7.1267, -8.1869) -> (-7.6397, -8.1869)
  line L63 (-7.6397, -8.1869) -> (-7.6397, -9)
  line L64 (-7.6397, -9) -> (-7.9043, -9)
  line L65 (-7.6397, -7.9509) -> (-7.1226, -7.9509)
  spline S41 degree 2 poles (-7.1226, -7.9509) (-6.8661, -7.9509) (-6.7584, -7.8554) knots 0 0 0 1 1 1
  spline S42 degree 2 poles (-6.7584, -7.8554) (-6.6506, -7.7599) (-6.6506, -7.5866) knots 0 0 0 1 1 1
  spline S43 degree 2 poles (-6.6506, -7.5866) (-6.6506, -7.4611) (-6.7147, -7.3724) knots 0 0 0 1 1 1
  spline S44 degree 2 poles (-6.7147, -7.3724) (-6.7775, -7.2824) (-6.8811, -7.2538) knots 0 0 0 1 1 1
  spline S45 degree 2 poles (-6.8811, -7.2538) (-6.948, -7.236) (-7.1281, -7.236) knots 0 0 0 1 1 1
  line L66 (-7.1281, -7.236) -> (-7.6397, -7.236)
  line L67 (-7.6397, -7.236) -> (-7.6397, -7.9509)
  line L68 (-11.8245, -5.3574) -> (-11.5748, -5.3356)
  spline S46 degree 2 poles (-11.5748, -5.3356) (-11.5571, -5.4857) (-11.493, -5.5825) knots 0 0 0 1 1 1
  spline S47 degree 2 poles (-11.493, -5.5825) (-11.4275, -5.678) (-11.2911, -5.7381) knots 0 0 0 1 1 1
  spline S48 degree 2 poles (-11.2911, -5.7381) (-11.1546, -5.7967) (-10.9841, -5.7967) knots 0 0 0 1 1 1
  spline S49 degree 2 poles (-10.9841, -5.7967) (-10.8327, -5.7967) (-10.7167, -5.7517) knots 0 0 0 1 1 1
  spline S50 degree 2 poles (-10.7167, -5.7517) (-10.6008, -5.7067) (-10.5448, -5.6289) knots 0 0 0 1 1 1
  spline S51 degree 2 poles (-10.5448, -5.6289) (-10.4875, -5.5498) (-10.4875, -5.457) knots 0 0 0 1 1 1
  spline S52 degree 2 poles (-10.4875, -5.457) (-10.4875, -5.3629) (-10.5421, -5.2933) knots 0 0 0 1 1 1
  spline S53 degree 2 poles (-10.5421, -5.2933) (-10.5967, -5.2224) (-10.7222, -5.1746) knots 0 0 0 1 1 1
  spline S54 degree 2 poles (-10.7222, -5.1746) (-10.8027, -5.1432) (-11.0782, -5.0778) knots 0 0 0 1 1 1
  spline S55 degree 2 poles (-11.0782, -5.0778) (-11.3538, -5.0109) (-11.4643, -4.9523) knots 0 0 0 1 1 1
  spline S56 degree 2 poles (-11.4643, -4.9523) (-11.6076, -4.8772) (-11.6785, -4.7667) knots 0 0 0 1 1 1
  spline S57 degree 2 poles (-11.6785, -4.7667) (-11.7481, -4.6548) (-11.7481, -4.5171) knots 0 0 0 1 1 1
  spline S58 degree 2 poles (-11.7481, -4.5171) (-11.7481, -4.3656) (-11.6621, -4.2347) knots 0 0 0 1 1 1
  spline S59 degree 2 poles (-11.6621, -4.2347) (-11.5762, -4.1023) (-11.4111, -4.0341) knots 0 0 0 1 1 1
  spline S60 degree 2 poles (-11.4111, -4.0341) (-11.246, -3.9659) (-11.0441, -3.9659) knots 0 0 0 1 1 1
  spline S61 degree 2 poles (-11.0441, -3.9659) (-10.8218, -3.9659) (-10.6526, -4.0382) knots 0 0 0 1 1 1
  spline S62 degree 2 poles (-10.6526, -4.0382) (-10.4821, -4.1091) (-10.3907, -4.2483) knots 0 0 0 1 1 1
  spline S63 degree 2 poles (-10.3907, -4.2483) (-10.2993, -4.3874) (-10.2924, -4.5634) knots 0 0 0 1 1 1
  line L69 (-10.2924, -4.5634) -> (-10.5462, -4.5825)
  spline S64 degree 2 poles (-10.5462, -4.5825) (-10.5666, -4.3929) (-10.6853, -4.296) knots 0 0 0 1 1 1
  spline S65 degree 2 poles (-10.6853, -4.296) (-10.8027, -4.1992) (-11.0332, -4.1992) knots 0 0 0 1 1 1
  spline S66 degree 2 poles (-11.0332, -4.1992) (-11.2733, -4.1992) (-11.3838, -4.2879) knots 0 0 0 1 1 1
  spline S67 degree 2 poles (-11.3838, -4.2879) (-11.493, -4.3752) (-11.493, -4.4993) knots 0 0 0 1 1 1
  spline S68 degree 2 poles (-11.493, -4.4993) (-11.493, -4.6071) (-11.4152, -4.6767) knots 0 0 0 1 1 1
  spline S69 degree 2 poles (-11.4152, -4.6767) (-11.3388, -4.7462) (-11.0168, -4.8199) knots 0 0 0 1 1 1
  spline S70 degree 2 poles (-11.0168, -4.8199) (-10.6935, -4.8922) (-10.5735, -4.9468) knots 0 0 0 1 1 1
  spline S71 degree 2 poles (-10.5735, -4.9468) (-10.3988, -5.0273) (-10.3156, -5.1514) knots 0 0 0 1 1 1
  spline S72 degree 2 poles (-10.3156, -5.1514) (-10.2324, -5.2742) (-10.2324, -5.4352) knots 0 0 0 1 1 1
  spline S73 degree 2 poles (-10.2324, -5.4352) (-10.2324, -5.5948) (-10.3238, -5.7367) knots 0 0 0 1 1 1
  spline S74 degree 2 poles (-10.3238, -5.7367) (-10.4152, -5.8772) (-10.5871, -5.9563) knots 0 0 0 1 1 1
  spline S75 degree 2 poles (-10.5871, -5.9563) (-10.7576, -6.0341) (-10.9718, -6.0341) knots 0 0 0 1 1 1
  spline S76 degree 2 poles (-10.9718, -6.0341) (-11.2433, -6.0341) (-11.4275, -5.955) knots 0 0 0 1 1 1
  spline S77 degree 2 poles (-11.4275, -5.955) (-11.6103, -5.8759) (-11.7153, -5.7176) knots 0 0 0 1 1 1
  spline S78 degree 2 poles (-11.7153, -5.7176) (-11.819, -5.558) (-11.8245, -5.3574) knots 0 0 0 1 1 1
  line L70 (-9.5216, -6) -> (-10.0523, -4)
  line L71 (-10.0523, -4) -> (-9.7808, -4)
  line L72 (-9.7808, -4) -> (-9.4766, -5.3111)
  spline S79 degree 2 poles (-9.4766, -5.3111) (-9.4275, -5.5171) (-9.392, -5.7203) knots 0 0 0 1 1 1
  spline S80 degree 2 poles (-9.392, -5.7203) (-9.3156, -5.3997) (-9.302, -5.3506) knots 0 0 0 1 1 1
  line L73 (-9.302, -5.3506) -> (-8.9214, -4)
  line L74 (-8.9214, -4) -> (-8.6021, -4)
  line L75 (-8.6021, -4) -> (-8.3156, -5.0123)
  spline S81 degree 2 poles (-8.3156, -5.0123) (-8.2078, -5.3888) (-8.1601, -5.7203) knots 0 0 0 1 1 1
  spline S82 degree 2 poles (-8.1601, -5.7203) (-8.1219, -5.5307) (-8.0605, -5.2851) knots 0 0 0 1 1 1
  line L76 (-8.0605, -5.2851) -> (-7.7467, -4)
  line L77 (-7.7467, -4) -> (-7.4807, -4)
  line L78 (-7.4807, -4) -> (-8.0291, -6)
  line L79 (-8.0291, -6) -> (-8.2842, -6)
  line L80 (-8.2842, -6) -> (-8.7058, -4.4761)
  spline S83 degree 2 poles (-8.7058, -4.4761) (-8.759, -4.2851) (-8.7686, -4.2415) knots 0 0 0 1 1 1
  spline S84 degree 2 poles (-8.7686, -4.2415) (-8.7999, -4.3793) (-8.8272, -4.4761) knots 0 0 0 1 1 1
  line L81 (-8.8272, -4.4761) -> (-9.2515, -6)
  line L82 (-9.2515, -6) -> (-9.5216, -6)
  line L83 (2.596, -8.472) -> (2.8416, -8.4393)
  spline S85 degree 2 poles (2.8416, -8.4393) (2.8839, -8.648) (2.9848, -8.7408) knots 0 0 0 1 1 1
  spline S86 degree 2 poles (2.9848, -8.7408) (3.0871, -8.8322) (3.2331, -8.8322) knots 0 0 0 1 1 1
  spline S87 degree 2 poles (3.2331, -8.8322) (3.4064, -8.8322) (3.5251, -8.7121) knots 0 0 0 1 1 1
  spline S88 degree 2 poles (3.5251, -8.7121) (3.6451, -8.5921) (3.6451, -8.4147) knots 0 0 0 1 1 1
  spline S89 degree 2 poles (3.6451, -8.4147) (3.6451, -8.2456) (3.5346, -8.1364) knots 0 0 0 1 1 1
  spline S90 degree 2 poles (3.5346, -8.1364) (3.4241, -8.0259) (3.2536, -8.0259) knots 0 0 0 1 1 1
  spline S91 degree 2 poles (3.2536, -8.0259) (3.184, -8.0259) (3.0803, -8.0532) knots 0 0 0 1 1 1
  line L84 (3.0803, -8.0532) -> (3.1076, -7.8377)
  spline S92 degree 2 poles (3.1076, -7.8377) (3.1322, -7.8404) (3.1472, -7.8404) knots 0 0 0 1 1 1
  spline S93 degree 2 poles (3.1472, -7.8404) (3.3041, -7.8404) (3.4296, -7.7585) knots 0 0 0 1 1 1
  spline S94 degree 2 poles (3.4296, -7.7585) (3.5551, -7.6767) (3.5551, -7.5061) knots 0 0 0 1 1 1
  spline S95 degree 2 poles (3.5551, -7.5061) (3.5551, -7.3711) (3.4637, -7.2824) knots 0 0 0 1 1 1
  spline S96 degree 2 poles (3.4637, -7.2824) (3.3723, -7.1937) (3.2277, -7.1937) knots 0 0 0 1 1 1
  spline S97 degree 2 poles (3.2277, -7.1937) (3.0844, -7.1937) (2.9889, -7.2838) knots 0 0 0 1 1 1
  spline S98 degree 2 poles (2.9889, -7.2838) (2.8934, -7.3738) (2.8661, -7.5539) knots 0 0 0 1 1 1
  line L85 (2.8661, -7.5539) -> (2.6206, -7.5102)
  spline S99 degree 2 poles (2.6206, -7.5102) (2.6656, -7.2633) (2.8252, -7.1282) knots 0 0 0 1 1 1
  spline S100 degree 2 poles (2.8252, -7.1282) (2.9848, -6.9918) (3.2222, -6.9918) knots 0 0 0 1 1 1
  spline S101 degree 2 poles (3.2222, -6.9918) (3.3859, -6.9918) (3.5237, -7.0628) knots 0 0 0 1 1 1
  spline S102 degree 2 poles (3.5237, -7.0628) (3.6615, -7.1323) (3.7338, -7.2538) knots 0 0 0 1 1 1
  spline S103 degree 2 poles (3.7338, -7.2538) (3.8075, -7.3752) (3.8075, -7.5116) knots 0 0 0 1 1 1
  spline S104 degree 2 poles (3.8075, -7.5116) (3.8075, -7.6412) (3.7379, -7.7476) knots 0 0 0 1 1 1
  spline S105 degree 2 poles (3.7379, -7.7476) (3.6683, -7.854) (3.5319, -7.9168) knots 0 0 0 1 1 1
  spline S106 degree 2 poles (3.5319, -7.9168) (3.7092, -7.9577) (3.8075, -8.0873) knots 0 0 0 1 1 1
  spline S107 degree 2 poles (3.8075, -8.0873) (3.9057, -8.2156) (3.9057, -8.4093) knots 0 0 0 1 1 1
  spline S108 degree 2 poles (3.9057, -8.4093) (3.9057, -8.6712) (3.7147, -8.854) knots 0 0 0 1 1 1
  spline S109 degree 2 poles (3.7147, -8.854) (3.5237, -9.0355) (3.2318, -9.0355) knots 0 0 0 1 1 1
  spline S110 degree 2 poles (3.2318, -9.0355) (2.9685, -9.0355) (2.7938, -8.8786) knots 0 0 0 1 1 1
  spline S111 degree 2 poles (2.7938, -8.8786) (2.6206, -8.7217) (2.596, -8.472) knots 0 0 0 1 1 1
  spline S112 degree 2 poles (4.1485, -8.0136) (4.1485, -7.6589) (4.2208, -7.4434) knots 0 0 0 1 1 1
  spline S113 degree 2 poles (4.2208, -7.4434) (4.2945, -7.2265) (4.4378, -7.1091) knots 0 0 0 1 1 1
  spline S114 degree 2 poles (4.4378, -7.1091) (4.5824, -6.9918) (4.8006, -6.9918) knots 0 0 0 1 1 1
  spline S115 degree 2 poles (4.8006, -6.9918) (4.9616, -6.9918) (5.083, -7.0573) knots 0 0 0 1 1 1
  spline S116 degree 2 poles (5.083, -7.0573) (5.2045, -7.1214) (5.2836, -7.2442) knots 0 0 0 1 1 1
  spline S117 degree 2 poles (5.2836, -7.2442) (5.3627, -7.3656) (5.4077, -7.5416) knots 0 0 0 1 1 1
  spline S118 degree 2 poles (5.4077, -7.5416) (5.4528, -7.7162) (5.4528, -8.0136) knots 0 0 0 1 1 1
  spline S119 degree 2 poles (5.4528, -8.0136) (5.4528, -8.3656) (5.3805, -8.5825) knots 0 0 0 1 1 1
  spline S120 degree 2 poles (5.3805, -8.5825) (5.3082, -8.7981) (5.1635, -8.9168) knots 0 0 0 1 1 1
  spline S121 degree 2 poles (5.1635, -8.9168) (5.0203, -9.0341) (4.8006, -9.0341) knots 0 0 0 1 1 1
  spline S122 degree 2 poles (4.8006, -9.0341) (4.5114, -9.0341) (4.3464, -8.8267) knots 0 0 0 1 1 1
  spline S123 degree 2 poles (4.3464, -8.8267) (4.1485, -8.5771) (4.1485, -8.0136) knots 0 0 0 1 1 1
  spline S124 degree 2 poles (4.4009, -8.0136) (4.4009, -8.5061) (4.5155, -8.6698) knots 0 0 0 1 1 1
  spline S125 degree 2 poles (4.5155, -8.6698) (4.6315, -8.8322) (4.8006, -8.8322) knots 0 0 0 1 1 1
  spline S126 degree 2 poles (4.8006, -8.8322) (4.9698, -8.8322) (5.0844, -8.6685) knots 0 0 0 1 1 1
  spline S127 degree 2 poles (5.0844, -8.6685) (5.2004, -8.5048) (5.2004, -8.0136) knots 0 0 0 1 1 1
  spline S128 degree 2 poles (5.2004, -8.0136) (5.2004, -7.5198) (5.0844, -7.3574) knots 0 0 0 1 1 1
  spline S129 degree 2 poles (5.0844, -7.3574) (4.9698, -7.1951) (4.7979, -7.1951) knots 0 0 0 1 1 1
  spline S130 degree 2 poles (4.7979, -7.1951) (4.6288, -7.1951) (4.5278, -7.3383) knots 0 0 0 1 1 1
  spline S131 degree 2 poles (4.5278, -7.3383) (4.4009, -7.5211) (4.4009, -8.0136) knots 0 0 0 1 1 1
  line L86 (6.3736, -9) -> (5.5987, -7)
  line L87 (5.5987, -7) -> (5.8852, -7)
  line L88 (5.8852, -7) -> (6.405, -8.4529)
  spline S132 degree 2 poles (6.405, -8.4529) (6.4678, -8.6276) (6.5101, -8.7804) knots 0 0 0 1 1 1
  spline S133 degree 2 poles (6.5101, -8.7804) (6.5564, -8.6166) (6.6178, -8.4529) knots 0 0 0 1 1 1
  line L89 (6.6178, -8.4529) -> (7.1581, -7)
  line L90 (7.1581, -7) -> (7.4282, -7)
  line L91 (7.4282, -7) -> (6.6451, -9)
  line L92 (6.6451, -9) -> (6.3736, -9)
  line L93 (7.6656, -9) -> (7.6656, -7)
  line L94 (7.6656, -7) -> (8.3545, -7)
  spline S134 degree 2 poles (8.3545, -7) (8.5878, -7) (8.7106, -7.0286) knots 0 0 0 1 1 1
  spline S135 degree 2 poles (8.7106, -7.0286) (8.8825, -7.0682) (9.0039, -7.1719) knots 0 0 0 1 1 1
  spline S136 degree 2 poles (9.0039, -7.1719) (9.1622, -7.3056) (9.2399, -7.5143) knots 0 0 0 1 1 1
  spline S137 degree 2 poles (9.2399, -7.5143) (9.3191, -7.7217) (9.3191, -7.9891) knots 0 0 0 1 1 1
  spline S138 degree 2 poles (9.3191, -7.9891) (9.3191, -8.2169) (9.2659, -8.3929) knots 0 0 0 1 1 1
  spline S139 degree 2 poles (9.2659, -8.3929) (9.2127, -8.5689) (9.1294, -8.6849) knots 0 0 0 1 1 1
  spline S140 degree 2 poles (9.1294, -8.6849) (9.0462, -8.7995) (8.9466, -8.8663) knots 0 0 0 1 1 1
  spline S141 degree 2 poles (8.9466, -8.8663) (8.8484, -8.9318) (8.7079, -8.9659) knots 0 0 0 1 1 1
  spline S142 degree 2 poles (8.7079, -8.9659) (8.5687, -9) (8.3873, -9) knots 0 0 0 1 1 1
  line L95 (8.3873, -9) -> (7.6656, -9)
  line L96 (7.9303, -8.764) -> (8.3573, -8.764)
  spline S143 degree 2 poles (8.3573, -8.764) (8.5551, -8.764) (8.667, -8.7271) knots 0 0 0 1 1 1
  spline S144 degree 2 poles (8.667, -8.7271) (8.7802, -8.6903) (8.847, -8.6235) knots 0 0 0 1 1 1
  spline S145 degree 2 poles (8.847, -8.6235) (8.9412, -8.5293) (8.993, -8.3711) knots 0 0 0 1 1 1
  spline S146 degree 2 poles (8.993, -8.3711) (9.0462, -8.2115) (9.0462, -7.985) knots 0 0 0 1 1 1
  spline S147 degree 2 poles (9.0462, -7.985) (9.0462, -7.6712) (8.9425, -7.5034) knots 0 0 0 1 1 1
  spline S148 degree 2 poles (8.9425, -7.5034) (8.8402, -7.3342) (8.6929, -7.2769) knots 0 0 0 1 1 1
  spline S149 degree 2 poles (8.6929, -7.2769) (8.5865, -7.236) (8.3504, -7.236) knots 0 0 0 1 1 1
  line L97 (8.3504, -7.236) -> (7.9303, -7.236)
  line L98 (7.9303, -7.236) -> (7.9303, -8.764)
  line L99 (11.1103, -8.2988) -> (11.375, -8.3656)
  spline S150 degree 2 poles (11.375, -8.3656) (11.2918, -8.6917) (11.0749, -8.8636) knots 0 0 0 1 1 1
  spline S151 degree 2 poles (11.0749, -8.8636) (10.8593, -9.0341) (10.5469, -9.0341) knots 0 0 0 1 1 1
  spline S152 degree 2 poles (10.5469, -9.0341) (10.2236, -9.0341) (10.0203, -8.9031) knots 0 0 0 1 1 1
  spline S153 degree 2 poles (10.0203, -8.9031) (9.8184, -8.7708) (9.712, -8.5211) knots 0 0 0 1 1 1
  spline S154 degree 2 poles (9.712, -8.5211) (9.6069, -8.2715) (9.6069, -7.985) knots 0 0 0 1 1 1
  spline S155 degree 2 poles (9.6069, -7.985) (9.6069, -7.6726) (9.7256, -7.4407) knots 0 0 0 1 1 1
  spline S156 degree 2 poles (9.7256, -7.4407) (9.8457, -7.2074) (10.0653, -7.0873) knots 0 0 0 1 1 1
  spline S157 degree 2 poles (10.0653, -7.0873) (10.2863, -6.9659) (10.551, -6.9659) knots 0 0 0 1 1 1
  spline S158 degree 2 poles (10.551, -6.9659) (10.8511, -6.9659) (11.0558, -7.1187) knots 0 0 0 1 1 1
  spline S159 degree 2 poles (11.0558, -7.1187) (11.2604, -7.2715) (11.3409, -7.5484) knots 0 0 0 1 1 1
  line L100 (11.3409, -7.5484) -> (11.0803, -7.6098)
  spline S160 degree 2 poles (11.0803, -7.6098) (11.0107, -7.3915) (10.8784, -7.292) knots 0 0 0 1 1 1
  spline S161 degree 2 poles (10.8784, -7.292) (10.7461, -7.1924) (10.5455, -7.1924) knots 0 0 0 1 1 1
  spline S162 degree 2 poles (10.5455, -7.1924) (10.315, -7.1924) (10.1594, -7.3029) knots 0 0 0 1 1 1
  spline S163 degree 2 poles (10.1594, -7.3029) (10.0053, -7.4134) (9.9425, -7.6003) knots 0 0 0 1 1 1
  spline S164 degree 2 poles (9.9425, -7.6003) (9.8798, -7.7858) (9.8798, -7.9836) knots 0 0 0 1 1 1
  spline S165 degree 2 poles (9.8798, -7.9836) (9.8798, -8.2387) (9.9534, -8.4297) knots 0 0 0 1 1 1
  spline S166 degree 2 poles (9.9534, -8.4297) (10.0285, -8.6194) (10.1854, -8.7135) knots 0 0 0 1 1 1
  spline S167 degree 2 poles (10.1854, -8.7135) (10.3423, -8.8076) (10.5251, -8.8076) knots 0 0 0 1 1 1
  spline S168 degree 2 poles (10.5251, -8.8076) (10.7474, -8.8076) (10.9016, -8.6794) knots 0 0 0 1 1 1
  spline S169 degree 2 poles (10.9016, -8.6794) (11.0558, -8.5512) (11.1103, -8.2988) knots 0 0 0 1 1 1
  line L101 (-11.0496, -3) -> (-11.8245, -1)
  line L102 (-11.8245, -1) -> (-11.538, -1)
  line L103 (-11.538, -1) -> (-11.0182, -2.4529)
  spline S170 degree 2 poles (-11.0182, -2.4529) (-10.9555, -2.6276) (-10.9132, -2.7804) knots 0 0 0 1 1 1
  spline S171 degree 2 poles (-10.9132, -2.7804) (-10.8668, -2.6166) (-10.8054, -2.4529) knots 0 0 0 1 1 1
  line L104 (-10.8054, -2.4529) -> (-10.2651, -1)
  line L105 (-10.2651, -1) -> (-9.995, -1)
  line L106 (-9.995, -1) -> (-10.7781, -3)
  line L107 (-10.7781, -3) -> (-11.0496, -3)
  line L108 (-9.8845, -2.3997) -> (-9.8845, -2.1528)
  line L109 (-9.8845, -2.1528) -> (-9.1301, -2.1528)
  line L110 (-9.1301, -2.1528) -> (-9.1301, -2.3997)
  line L111 (-9.1301, -2.3997) -> (-9.8845, -2.3997)
  line L112 (-8.0018, -3) -> (-8.2474, -3)
  line L113 (-8.2474, -3) -> (-8.2474, -1.4352)
  spline S172 degree 2 poles (-8.2474, -1.4352) (-8.3361, -1.5198) (-8.4807, -1.6044) knots 0 0 0 1 1 1
  spline S173 degree 2 poles (-8.4807, -1.6044) (-8.6239, -1.6889) (-8.7385, -1.7312) knots 0 0 0 1 1 1
  line L114 (-8.7385, -1.7312) -> (-8.7385, -1.4939)
  spline S174 degree 2 poles (-8.7385, -1.4939) (-8.5325, -1.397) (-8.3784, -1.2592) knots 0 0 0 1 1 1
  spline S175 degree 2 poles (-8.3784, -1.2592) (-8.2242, -1.1214) (-8.1601, -0.9918) knots 0 0 0 1 1 1
  line L115 (-8.1601, -0.9918) -> (-8.0018, -0.9918)
  line L116 (-8.0018, -0.9918) -> (-8.0018, -3)
  line L117 (-6.448, -3) -> (-6.6935, -3)
  line L118 (-6.6935, -3) -> (-6.6935, -1.4352)
  spline S176 degree 2 poles (-6.6935, -1.4352) (-6.7822, -1.5198) (-6.9268, -1.6044) knots 0 0 0 1 1 1
  spline S177 degree 2 poles (-6.9268, -1.6044) (-7.0701, -1.6889) (-7.1847, -1.7312) knots 0 0 0 1 1 1
  line L119 (-7.1847, -1.7312) -> (-7.1847, -1.4939)
  spline S178 degree 2 poles (-7.1847, -1.4939) (-6.9787, -1.397) (-6.8245, -1.2592) knots 0 0 0 1 1 1
  spline S179 degree 2 poles (-6.8245, -1.2592) (-6.6703, -1.1214) (-6.6062, -0.9918) knots 0 0 0 1 1 1
  line L120 (-6.6062, -0.9918) -> (-6.448, -0.9918)
  line L121 (-6.448, -0.9918) -> (-6.448, -3)
  line L122 (-5.8463, -2.3997) -> (-5.8463, -2.1528)
  line L123 (-5.8463, -2.1528) -> (-5.0919, -2.1528)
  line L124 (-5.0919, -2.1528) -> (-5.0919, -2.3997)
  line L125 (-5.0919, -2.3997) -> (-5.8463, -2.3997)
  line L126 (-4.8872, -2.472) -> (-4.6417, -2.4393)
  spline S180 degree 2 poles (-4.6417, -2.4393) (-4.5994, -2.648) (-4.4984, -2.7408) knots 0 0 0 1 1 1
  spline S181 degree 2 poles (-4.4984, -2.7408) (-4.3961, -2.8322) (-4.2501, -2.8322) knots 0 0 0 1 1 1
  spline S182 degree 2 poles (-4.2501, -2.8322) (-4.0769, -2.8322) (-3.9582, -2.7121) knots 0 0 0 1 1 1
  spline S183 degree 2 poles (-3.9582, -2.7121) (-3.8381, -2.5921) (-3.8381, -2.4147) knots 0 0 0 1 1 1
  spline S184 degree 2 poles (-3.8381, -2.4147) (-3.8381, -2.2456) (-3.9486, -2.1364) knots 0 0 0 1 1 1
  spline S185 degree 2 poles (-3.9486, -2.1364) (-4.0591, -2.0259) (-4.2297, -2.0259) knots 0 0 0 1 1 1
  spline S186 degree 2 poles (-4.2297, -2.0259) (-4.2993, -2.0259) (-4.4029, -2.0532) knots 0 0 0 1 1 1
  line L127 (-4.4029, -2.0532) -> (-4.3756, -1.8377)
  spline S187 degree 2 poles (-4.3756, -1.8377) (-4.3511, -1.8404) (-4.3361, -1.8404) knots 0 0 0 1 1 1
  spline S188 degree 2 poles (-4.3361, -1.8404) (-4.1792, -1.8404) (-4.0537, -1.7585) knots 0 0 0 1 1 1
  spline S189 degree 2 poles (-4.0537, -1.7585) (-3.9282, -1.6767) (-3.9282, -1.5061) knots 0 0 0 1 1 1
  spline S190 degree 2 poles (-3.9282, -1.5061) (-3.9282, -1.3711) (-4.0196, -1.2824) knots 0 0 0 1 1 1
  spline S191 degree 2 poles (-4.0196, -1.2824) (-4.111, -1.1937) (-4.2556, -1.1937) knots 0 0 0 1 1 1
  spline S192 degree 2 poles (-4.2556, -1.1937) (-4.3988, -1.1937) (-4.4943, -1.2838) knots 0 0 0 1 1 1
  spline S193 degree 2 poles (-4.4943, -1.2838) (-4.5898, -1.3738) (-4.6171, -1.5539) knots 0 0 0 1 1 1
  line L128 (-4.6171, -1.5539) -> (-4.8627, -1.5102)
  spline S194 degree 2 poles (-4.8627, -1.5102) (-4.8177, -1.2633) (-4.6581, -1.1282) knots 0 0 0 1 1 1
  spline S195 degree 2 poles (-4.6581, -1.1282) (-4.4984, -0.9918) (-4.2611, -0.9918) knots 0 0 0 1 1 1
  spline S196 degree 2 poles (-4.2611, -0.9918) (-4.0973, -0.9918) (-3.9596, -1.0628) knots 0 0 0 1 1 1
  spline S197 degree 2 poles (-3.9596, -1.0628) (-3.8218, -1.1323) (-3.7495, -1.2538) knots 0 0 0 1 1 1
  spline S198 degree 2 poles (-3.7495, -1.2538) (-3.6758, -1.3752) (-3.6758, -1.5116) knots 0 0 0 1 1 1
  spline S199 degree 2 poles (-3.6758, -1.5116) (-3.6758, -1.6412) (-3.7454, -1.7476) knots 0 0 0 1 1 1
  spline S200 degree 2 poles (-3.7454, -1.7476) (-3.8149, -1.854) (-3.9514, -1.9168) knots 0 0 0 1 1 1
  spline S201 degree 2 poles (-3.9514, -1.9168) (-3.774, -1.9577) (-3.6758, -2.0873) knots 0 0 0 1 1 1
  spline S202 degree 2 poles (-3.6758, -2.0873) (-3.5776, -2.2156) (-3.5776, -2.4093) knots 0 0 0 1 1 1